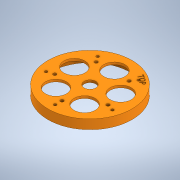
# Autodesk Inventor part: filterHolder
Saved by Autodesk Inventor 2022.1 (Build 261234000, 234)
## iProperties
Created: 2020-04-12
Part Number: filterHolder
Material: PBT Plastic
Document SubType Name: Modeling
Designer: robst
Density: 1.31 g/cm^3
Appearance: Orange
wheelOuterDiameter: 4.501 in
wheelFilterDiameter: 2.611 in
filterThreadDiameter: 1.125 in
numberOfFilters: 5.000 ul
d5: 360.00 deg
distanceBetweenFilters: 0.500 in
distanceFromFilterToEdge: 0.375 in
wheelFilterCircumference: 8.200 in
filterDiameter: 1.140 in
Author: robst
Autodesk Inventor part; units mm, degrees
ref_plane "YZ Plane" through (0, 0, 0) normal (1, 0, 0) x (0, 1, 0)
ref_plane "XZ Plane" through (0, 0, 0) normal (0, 1, 0) x (-1, 0, 0)
ref_plane "XY Plane" through (0, 0, 0) normal (0, 0, 1) x (1, 0, 0)
sketch "Sketch1" plane through (0, 0, 0) normal (0, 1, 0) x (-1, 0, 0)
  circle A0 centre (0, 0) radius 57.1686
  circle A1 centre (0, 0) radius 33.1656 construction
  circle A2 centre (0, -33.1656) radius 14.2875
  circle A3 centre (31.5424, -10.2487) radius 14.2875
  circle A4 centre (19.4943, 26.8315) radius 14.2875
  circle A5 centre (-19.4943, 26.8315) radius 14.2875
  circle A6 centre (-31.5424, -10.2487) radius 14.2875
  dimension "wheelFilterDiameter" = 66.3312
  dimension "wheelOuterDiameter" = 114.3372
  dimension "filterThreadDiameter" = 28.575
  dimension "d5" = 360
  constraints: 6 centre point, 2 coincident, 1 vertical alignment, 13 other
  measures "wheelOuterDiameter" diameter of A0
  measures "filterThreadDiameter" diameter of A2
extrude "Extrusion5" add sketch "Sketch1" against normal blind 3.175
sketch "Sketch5" plane through (0, 0, 0) normal (0, 1, 0) x (1, 0, 0)
  arc A0 (35.921, 35.921) -> (0, 50.8) centre (0, 0) ccw construction
  line L0 (0, 50.8) -> (0, -50.8) construction
  line L1 (50.8, 0) -> (-50.8, 0) construction
  line L2 (0, 0) -> (35.921, 35.921) construction
  line L3 (23.0912, 41.7997) -> (25.7305, 46.4819)
  line L4 (25.7305, 46.4819) -> (23.9488, 47.4861)
  line L5 (23.9488, 47.4861) -> (24.303, 48.1144)
  line L6 (24.303, 48.1144) -> (28.572, 45.7081)
  line L7 (28.572, 45.7081) -> (28.2178, 45.0798)
  line L8 (28.2178, 45.0798) -> (26.4362, 46.084)
  line L9 (26.4362, 46.084) -> (23.797, 41.4019)
  line L10 (23.797, 41.4019) -> (23.0912, 41.7997)
  spline S0 degree 2 poles (32.7583, 41.9026) (32.8009, 41.3717) (32.4178, 40.1854) (31.9717, 39.5691) knots 0 0 0 1 2 2 2
  spline S1 degree 2 poles (31.9717, 39.5691) (31.5371, 38.9689) (30.5291, 38.2167) (30.0034, 38.0971) knots 0 0 0 1 2 2 2
  spline S2 degree 2 poles (30.0034, 38.0971) (29.4502, 37.9731) (28.4083, 38.2273) (27.9242, 38.5778) knots 0 0 0 1 2 2 2
  spline S3 degree 2 poles (27.9242, 38.5778) (27.424, 38.9399) (26.8699, 39.8594) (26.8182, 40.403) knots 0 0 0 1 2 2 2
  spline S4 degree 2 poles (26.8182, 40.403) (26.7716, 40.9368) (27.1656, 42.1213) (27.606, 42.7295) knots 0 0 0 1 2 2 2
  spline S5 degree 2 poles (27.606, 42.7295) (28.055, 43.3498) (29.0467, 44.0711) (29.5771, 44.2055) knots 0 0 0 1 2 2 2
  spline S6 degree 2 poles (29.5771, 44.2055) (30.1027, 44.3251) (31.1533, 44.083) (31.6495, 43.7238) knots 0 0 0 1 2 2 2
  spline S7 degree 2 poles (31.6495, 43.7238) (32.1536, 43.3588) (32.707, 42.4215) (32.7583, 41.9026) knots 0 0 0 1 2 2 2
  spline S8 degree 2 poles (31.2874, 40.0645) (31.6408, 40.5527) (31.9762, 41.4625) (31.9637, 41.8496) knots 0 0 0 1 2 2 2
  spline S9 degree 2 poles (31.9637, 41.8496) (31.9531, 42.2477) (31.5862, 42.9035) (31.2421, 43.1527) knots 0 0 0 1 2 2 2
  spline S10 degree 2 poles (31.2421, 43.1527) (30.886, 43.4105) (30.1702, 43.5505) (29.7749, 43.4342) knots 0 0 0 1 2 2 2
  spline S11 degree 2 poles (29.7749, 43.4342) (29.3963, 43.324) (28.6378, 42.7144) (28.2902, 42.2342) knots 0 0 0 1 2 2 2
  spline S12 degree 2 poles (28.2902, 42.2342) (27.5863, 41.2618) (27.6552, 39.6385) (28.3395, 39.1431) knots 0 0 0 1 2 2 2
  spline S13 degree 2 poles (28.3395, 39.1431) (29.0238, 38.6477) (30.5835, 39.0921) (31.2874, 40.0645) knots 0 0 0 1 2 2 2
  spline S14 degree 2 poles (36.5539, 37.0614) (36.2883, 36.7688) (35.6016, 36.4313) (35.2491, 36.4177) knots 0 0 0 1 2 2 2
  spline S15 degree 2 poles (35.2491, 36.4177) (34.8058, 36.3997) (33.9572, 36.7363) (33.4743, 37.1746) knots 0 0 0 1 2 2 2
  line L11 (33.4743, 37.1746) -> (32.9659, 37.6361)
  line L12 (32.9659, 37.6361) -> (31.4386, 35.9534)
  line L13 (31.4386, 35.9534) -> (30.8387, 36.4979)
  line L14 (30.8387, 36.4979) -> (34.9357, 41.0119)
  line L15 (34.9357, 41.0119) -> (36.0697, 39.9826)
  spline S16 degree 2 poles (36.0697, 39.9826) (36.4721, 39.6174) (36.9159, 38.9744) (36.9956, 38.6286) knots 0 0 0 1 2 2 2
  spline S17 degree 2 poles (36.9956, 38.6286) (37.0919, 38.2276) (36.8958, 37.4382) (36.5539, 37.0614) knots 0 0 0 1 2 2 2
  spline S18 degree 2 poles (35.9117, 37.6109) (36.1242, 37.845) (36.2754, 38.3349) (36.2104, 38.594) knots 0 0 0 1 2 2 2
  spline S19 degree 2 poles (36.2104, 38.594) (36.154, 38.8186) (35.8433, 39.2407) (35.5617, 39.4964) knots 0 0 0 1 2 2 2
  line L16 (35.5617, 39.4964) -> (35.0642, 39.9479)
  line L17 (35.0642, 39.9479) -> (33.4307, 38.1482)
  line L18 (33.4307, 38.1482) -> (33.8404, 37.7764)
  spline S20 degree 2 poles (33.8404, 37.7764) (34.2062, 37.4443) (34.7623, 37.153) (35.0481, 37.1739) knots 0 0 0 1 2 2 2
  spline S21 degree 2 poles (35.0481, 37.1739) (35.3063, 37.1864) (35.7159, 37.395) (35.9117, 37.6109) knots 0 0 0 1 2 2 2
  dimension "d25" = 101.6
  constraints: 6 end point, 2 point on circle, 1 centre point, 1 coincident, 1 perpendicular, 1 vertical, 1 other
  measures "d25" diameter of A0
extrude "Extrusion6" cut sketch "Sketch5" against normal blind 1.016
sketch "Sketch6" plane through (0, 0, 0) normal (0, 1, 0) x (1, 0, 0)
  circle A0 centre (0, 0) radius 7.9375
  dimension "d28" = 15.875
  constraints: 1 centre point, 1 coincident
  measures "d28" diameter of A0
extrude "Extrusion7" cut sketch "Sketch6" against normal through all
sketch "Sketch7" plane through (0, -3.175, 0) normal (0, -1, 0) x (1, 0, 0)
  point P0 (27.8922, -38.3904)
  point P1 (-27.8922, -38.3904)
  point P2 (-45.1306, 14.6638)
  point P3 (0, 47.4531)
  point P4 (45.1306, 14.6638)
hole "Hole1" at (27.8922, -3.175, -38.3904) at (-27.8922, -3.175, -38.3904) at (-45.1306, -3.175, 14.6638) at (0, -3.175, 47.4531) at (45.1306, -3.175, 14.6638) direction (0, 1, 0) diameter 3.7973 end through all
sketch "Sketch8" plane through (0, -3.175, 0) normal (0, -1, 0) x (1, 0, 0)
  circle A0 centre (0, 0) radius 57.1686
  circle A1 centre (0, 0) radius 54.6286
  dimension "d38" = 114.3372
  dimension "d39" = 2.54
  constraints: 2 centre point, 2 coincident
  measures "d38" diameter of A0
  measures "d39" radial gap between concentric circles of A1 A0
extrude "Extrusion8" add sketch "Sketch8" along normal blind 9.525
sketch "Sketch9" plane through (0, 0, 0) normal (0, 1, 0) x (1, 0, 0)
  circle A0 centre (0, 0) radius 7.9375 construction
  circle A1 centre (0, 0) radius 38.1 construction
  line L0 (0, 0) -> (38.1, 0) construction
  line L1 (0, 0) -> (36.2353, -11.7735) construction
  circle A2 centre (19.4943, -26.8315) radius 14.2875 construction
  circle A3 centre (31.5424, 10.2487) radius 14.2875 construction
  line L2 (36.2353, -11.7735) -> (38.0188, -2.4866) construction
  circle A4 centre (31.5424, 10.2487) radius 14.2875 construction
  line L3 (36.2353, -11.7735) -> (32.2194, -20.3352) construction
  point P0 (22.3946, 30.8235)
  point P1 (-22.3946, 30.8235)
  point P2 (-36.2353, -11.7735)
  point P3 (0, -38.1)
  dimension "d42" = 76.2
  dimension "d45" = 360
  dimension "d54" = 18
  constraints: 8 end point, 4 point on circle, 2 coincident, 1 centre point, 1 equal length, 1 horizontal, 10 other
  measures "d42" diameter of A1
  measures "d54" angle of L1 L0
hole "Hole2" at (36.2353, 0, 11.7735) at (22.3946, 0, -30.8235) at (-22.3946, 0, -30.8235) at (-36.2353, 0, 11.7735) at (0, 0, 38.1) direction (0, -1, 0) diameter 4.4958 end through all clearance for "Flat Head Machine Screw (82)" size "#8" standard "Ansi Unified Screw Threads"
equation "\"wheelFilterDiameter\" = 0.318471 * wheelFilterCircumference"
equation "\"wheelOuterDiameter\" = filterDiameter + wheelFilterDiameter + 2 * distanceFromFilterToEdge"
equation "\"d23\" = filterWheelThickness"
equation "\"d26\" = textDepth"
equation "\"d28\" = centerHoleDiameter"
equation "\"distanceBetweenFilters\" = 12.7"
equation "\"distanceFromFilterToEdge\" = 9.525"
equation "\"filterDiameter\" = 28.956"
equation "\"filterWheelThickness\" = 3.175"
equation "\"textDepth\" = 1.016"
equation "\"centerHoleDiameter\" = 15.875"
equation "\"wheelFilterCircumference\" = 208.28"
body "Solid3"
